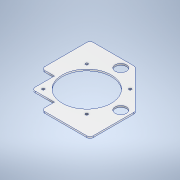
# Autodesk Inventor part: BottomPlate
Saved by Autodesk Inventor 2020 (Build 240168000, 168)
## iProperties
Created: 2019-05-28
Part Number: BottomPlate
Material: Aluminum 6061
Document SubType Name: Modeling
Designer: Connor
Density: 2.7 g/cm^3
Appearance: Aluminum - Flat
Author: Connor
Autodesk Inventor part; units mm, degrees
ref_plane "YZ Plane" through (0, 0, 0) normal (1, 0, 0) x (0, 1, 0)
ref_plane "XZ Plane" through (0, 0, 0) normal (0, 1, 0) x (-1, 0, 0)
ref_plane "XY Plane" through (0, 0, 0) normal (0, 0, 1) x (1, 0, 0)
sketch "Sketch1" plane through (0, 0, 0) normal (0, 1, 0) x (-1, 0, 0)
  line L0 (0, 0) -> (-165.1, 0)
  line L1 (-165.1, 0) -> (-165.1, -165.1)
  line L2 (-165.1, -165.1) -> (0, -165.1)
  line L3 (0, -165.1) -> (0, 0)
  circle A0 centre (-79.375, -79.375) radius 48.26
  line L4 (-25.4, -165.1) -> (-25.4, 0) construction
  line L5 (0, -25.4) -> (-165.1, -25.4) construction
  line L6 (0, 0) -> (-165.1, -165.1) construction
  circle A1 centre (-79.375, -79.375) radius 53.975 construction
  dimension "d0" = 96.52
  dimension "d3" = 25.4
  dimension "d4" = 25.4
  dimension "d5" = 107.95
  dimension "d24" = 165.1
  constraints: 14 end point, 7 point on line, 4 perpendicular, 2 centre point, 2 parallel, 1 coincident, 1 horizontal, 1 tangent
  measures "d0" diameter of A0
  measures "d3" distance between parallel lines of L0 L5
  measures "d4" distance between parallel lines of L3 L4
  measures "d5" diameter of A1
  measures "d24" distance between parallel lines of L0 L2
extrude "Extrusion1" add sketch "Sketch1" along normal blind 3.175
sketch "Sketch2" plane through (0, 3.175, 0) normal (0, 1, 0) x (1, 0, 0)
  circle A0 centre (79.375, 79.375) radius 48.26 construction
  circle A1 centre (79.375, 79.375) radius 60.325 construction
  line L0 (0, 165.1) -> (0, 0) construction
  arc A2 (177.8, 76.2) -> (76.2, 177.8) centre (76.2, 76.2) ccw construction
  line L1 (36.7188, 36.7188) -> (122.0312, 36.7188) construction
  line L2 (122.0312, 36.7188) -> (122.0312, 122.0312) construction
  line L3 (122.0312, 122.0312) -> (36.7188, 122.0312) construction
  line L4 (36.7188, 122.0312) -> (36.7188, 36.7188) construction
  dimension "d9" = 120.65
  constraints: 8 end point, 4 point on circle, 2 parallel, 2 perpendicular, 1 centre point, 1 coincident, 1 horizontal
  measures "d9" diameter of A1
hole "Hole1" at (36.7188, 3.175, -36.7188) at (122.0312, 3.175, -122.0312) at (122.0312, 3.175, -36.7188) at (36.7188, 3.175, -122.0312) direction (0, -1, 0) diameter 5.1594 end through all
sketch "Sketch4" plane through (0, 3.175, 0) normal (0, 1, 0) x (1, 0, 0)
  line L0 (0, 0) -> (165.1, 0) projected
  line L1 (0, 0) -> (25.4, 0)
  line L2 (25.4, 0) -> (25.4, 69.85)
  line L3 (25.4, 69.85) -> (0, 69.85)
  line L4 (0, 69.85) -> (0, 0)
  line L5 (25.4, 0) -> (69.85, 0)
  line L6 (69.85, 0) -> (69.85, 25.4)
  line L7 (69.85, 25.4) -> (25.4, 25.4)
  line L8 (25.4, 25.4) -> (25.4, 0)
  dimension "d26" = 25.4
  dimension "d27" = 69.85
  dimension "d28" = 44.45
  dimension "d29" = 25.4
  constraints: 16 end point, 4 parallel, 2 horizontal, 2 perpendicular
  measures "d26" distance of L3.end L2.end
  measures "d27" distance of L2.end L1.end
  measures "d28" distance of L7.end L6.end
  measures "d29" distance of L6.end L5.end
extrude "Extrusion3" cut sketch "Sketch4" against normal through all
chamfer "Chamfer1" distance 76.2 angle 45 1 edges at (165.1, 1.5875, -165.1)
fillet "Fillet4" radius 6.35 7 edges at (165.1, 1.5875, 0) (165.1, 1.5875, -88.9) (88.9, 1.5875, -165.1) (0, 1.5875, -165.1) (0, 1.5875, -69.85) (25.4, 1.5875, -25.4) (69.85, 1.5875, 0)
sketch "Sketch5" plane through (0, 3.175, 0) normal (0, 1, 0) x (1, 0, 0)
  circle A0 centre (148.6003, 77.0066) radius 11.1125
  circle A1 centre (79.375, 79.375) radius 48.26 construction
  circle A2 centre (79.375, 79.375) radius 69.2658 construction
  circle A3 centre (136.0149, 57.9229) radius 25.4 construction
  circle A4 centre (122.0312, 36.7188) radius 2.5797 construction
  circle A5 centre (136.0149, 57.9229) radius 22.86 construction
  line L0 (122.0312, 36.7188) -> (148.6003, 77.0066) construction
  circle A6 centre (36.7188, 36.7188) radius 2.5797 construction
  circle A7 centre (122.0312, 122.0312) radius 2.5797 construction
  line L1 (36.7188, 36.7188) -> (122.0312, 122.0312) construction
  circle A8 centre (77.0066, 148.6003) radius 11.1125
  point P0 (0, 0)
  dimension "d38" = 138.5316
  dimension "d39" = 50.8
  dimension "d40" = 45.72
  dimension "d37" = 22.225
  constraints: 4 end point, 2 centre point, 2 coincident, 1 point on line, 1 symmetric about line, 10 other
  measures "d37" diameter of A0
extrude "Extrusion4" cut sketch "Sketch5" against normal through all
body "Solid1"
